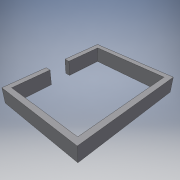
# Autodesk Inventor part: monitor frame part2 (for assembly)
Saved by Autodesk Inventor 2016 (Build 200138000, 138)
## iProperties
Created: 2017-10-23
Part Number: monitor frame part2 (for assembly)
Material: Generic
Document SubType Name: Modeling
Designer: student
Density: 1 g/cm^3
Appearance: Default
Author: student
Autodesk Inventor part; units mm, degrees
ref_plane "YZ Plane" through (0, 0, 0) normal (1, 0, 0) x (0, 1, 0)
ref_plane "XZ Plane" through (0, 0, 0) normal (0, 1, 0) x (-1, 0, 0)
ref_plane "XY Plane" through (0, 0, 0) normal (0, 0, 1) x (1, 0, 0)
sketch "Sketch1" plane through (0, 0, 0) normal (0, 1, 0) x (-1, 0, 0)
  line L0 (-203.2, 254) -> (203.2, 254)
  line L1 (203.2, 254) -> (203.2, -254)
  line L2 (203.2, -254) -> (-203.2, -254)
  line L3 (-203.2, -254) -> (-203.2, 254)
  line L4 (-203.2, 254) -> (203.2, -254) construction
  line L5 (203.2, 254) -> (-203.2, -254) construction
  point P0 (0, 0)
  dimension "d0" = 508
  dimension "d1" = 406.4
  constraints: 12 end point, 2 midpoint, 2 parallel, 1 horizontal, 1 perpendicular
  measures "d0" distance of L0.end L1.end
  measures "d1" distance of L1.end L2.end
extrude "Extrusion1" add sketch "Sketch1" along normal blind 71.12
sketch "Sketch2" plane through (0, 71.12, 0) normal (0, 1, 0) x (1, 0, 0)
  line L0 (177.8, -228.6) -> (-177.8, -228.6)
  line L1 (-177.8, -228.6) -> (-177.8, 228.6)
  line L2 (-177.8, 228.6) -> (177.8, 228.6)
  line L3 (177.8, 228.6) -> (177.8, -228.6)
  line L4 (177.8, -228.6) -> (-177.8, 228.6) construction
  line L5 (-177.8, -228.6) -> (177.8, 228.6) construction
  line L6 (-152.4, -50.8) -> (-203.2, -50.8)
  line L7 (-203.2, -50.8) -> (-203.2, 50.8)
  line L8 (-203.2, 50.8) -> (-152.4, 50.8)
  line L9 (-152.4, 50.8) -> (-152.4, -50.8)
  line L10 (-152.4, -50.8) -> (-203.2, 50.8) construction
  line L11 (-203.2, -50.8) -> (-152.4, 50.8) construction
  point P0 (0, 0)
  point P1 (-177.8, 0)
  dimension "d4" = 457.2
  dimension "d5" = 355.6
  dimension "d6" = 101.6
  constraints: 24 end point, 5 midpoint, 4 parallel, 2 horizontal, 2 perpendicular
  measures "d4" distance of L0.end L1.end
  measures "d5" distance of L1.end L2.end
  measures "d6" distance of L8.end L6.start
extrude "Extrusion2" cut sketch "Sketch2" against normal blind 71.12
body "Solid1"
